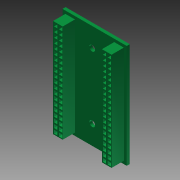
# Autodesk Inventor part: mbed breakout board
Saved by Autodesk Inventor 2012 (Build 160160000, 160)
## iProperties
Created: 2012-03-03
Part Number: mbed breakout board
Material: Default
Document SubType Name: Modeling
Designer: Lauszus
Density: 1 g/cm^3
Author: Lauszus
Autodesk Inventor part; units mm, degrees
ref_plane "YZ Plane" through (0, 0, 0) normal (1, 0, 0) x (0, 1, 0)
ref_plane "XZ Plane" through (0, 0, 0) normal (0, 1, 0) x (-1, 0, 0)
ref_plane "XY Plane" through (0, 0, 0) normal (0, 0, 1) x (1, 0, 0)
sketch "Sketch1" plane through (0, 0, 0) normal (0, 0, 1) x (1, 0, 0)
  line L0 (-20.4515, 31.3375) -> (12.9485, 31.3375)
  line L1 (12.9485, 31.3375) -> (12.9485, -22.6377)
  line L2 (12.9485, -22.6377) -> (-20.4515, -22.6377)
  line L3 (-20.4515, -22.6377) -> (-20.4515, 31.3375)
  line L4 (-18.9515, 29.8375) -> (-13.9515, 29.8375)
  line L5 (-13.9515, 29.8375) -> (-13.9515, -21.1377)
  line L6 (-13.9515, -21.1377) -> (-18.9515, -21.1377)
  line L7 (-18.9515, -21.1377) -> (-18.9515, 29.8375)
  line L8 (-18.4515, -20.6377) -> (-16.7515, -20.6377)
  line L9 (-16.7515, -20.6377) -> (-16.7515, -18.9377)
  line L10 (-16.7515, -18.9377) -> (-18.4515, -18.9377)
  line L11 (-18.4515, -18.9377) -> (-18.4515, -20.6377)
  line L12 (-15.9115, -20.6377) -> (-14.2115, -20.6377)
  line L13 (-14.2115, -20.6377) -> (-14.2115, -18.9377)
  line L14 (-14.2115, -18.9377) -> (-15.9115, -18.9377)
  line L15 (-15.9115, -18.9377) -> (-15.9115, -20.6377)
  line L16 (-18.4515, -18.0977) -> (-16.7515, -18.0977)
  line L17 (-16.7515, -18.0977) -> (-16.7515, -16.3977)
  line L18 (-16.7515, -16.3977) -> (-18.4515, -16.3977)
  line L19 (-18.4515, -16.3977) -> (-18.4515, -18.0977)
  line L20 (-15.9115, -18.0977) -> (-14.2115, -18.0977)
  line L21 (-14.2115, -18.0977) -> (-14.2115, -16.3977)
  line L22 (-14.2115, -16.3977) -> (-15.9115, -16.3977)
  line L23 (-15.9115, -16.3977) -> (-15.9115, -18.0977)
  line L24 (-18.4515, -15.5577) -> (-16.7515, -15.5577)
  line L25 (-16.7515, -15.5577) -> (-16.7515, -13.8577)
  line L26 (-16.7515, -13.8577) -> (-18.4515, -13.8577)
  line L27 (-18.4515, -13.8577) -> (-18.4515, -15.5577)
  line L28 (-15.9115, -15.5577) -> (-14.2115, -15.5577)
  line L29 (-14.2115, -15.5577) -> (-14.2115, -13.8577)
  line L30 (-14.2115, -13.8577) -> (-15.9115, -13.8577)
  line L31 (-15.9115, -13.8577) -> (-15.9115, -15.5577)
  line L32 (-14.2115, -11.3177) -> (-15.9115, -11.3177)
  line L33 (-14.2115, -13.0177) -> (-14.2115, -11.3177)
  line L34 (-15.9115, -11.3177) -> (-15.9115, -13.0177)
  line L35 (-15.9115, -13.0177) -> (-14.2115, -13.0177)
  line L36 (-18.4515, -13.0177) -> (-16.7515, -13.0177)
  line L37 (-16.7515, -13.0177) -> (-16.7515, -11.3177)
  line L38 (-16.7515, -11.3177) -> (-18.4515, -11.3177)
  line L39 (-18.4515, -11.3177) -> (-18.4515, -13.0177)
  line L40 (-18.4515, -10.4777) -> (-16.7515, -10.4777)
  line L41 (-16.7515, -10.4777) -> (-16.7515, -8.7777)
  line L42 (-16.7515, -8.7777) -> (-18.4515, -8.7777)
  line L43 (-18.4515, -8.7777) -> (-18.4515, -10.4777)
  line L44 (-15.9115, -10.4777) -> (-14.2115, -10.4777)
  line L45 (-14.2115, -10.4777) -> (-14.2115, -8.7777)
  line L46 (-14.2115, -8.7777) -> (-15.9115, -8.7777)
  line L47 (-15.9115, -8.7777) -> (-15.9115, -10.4777)
  line L48 (-14.2115, -6.2377) -> (-15.9115, -6.2377)
  line L49 (-14.2115, -7.9377) -> (-14.2115, -6.2377)
  line L50 (-15.9115, -6.2377) -> (-15.9115, -7.9377)
  line L51 (-15.9115, -7.9377) -> (-14.2115, -7.9377)
  line L52 (-18.4515, -7.9377) -> (-16.7515, -7.9377)
  line L53 (-16.7515, -7.9377) -> (-16.7515, -6.2377)
  line L54 (-16.7515, -6.2377) -> (-18.4515, -6.2377)
  line L55 (-18.4515, -6.2377) -> (-18.4515, -7.9377)
  line L56 (-18.4515, -5.3977) -> (-16.7515, -5.3977)
  line L57 (-16.7515, -5.3977) -> (-16.7515, -3.6977)
  line L58 (-16.7515, -3.6977) -> (-18.4515, -3.6977)
  line L59 (-18.4515, -3.6977) -> (-18.4515, -5.3977)
  line L60 (-15.9115, -5.3977) -> (-14.2115, -5.3977)
  line L61 (-14.2115, -5.3977) -> (-14.2115, -3.6977)
  line L62 (-14.2115, -3.6977) -> (-15.9115, -3.6977)
  line L63 (-15.9115, -3.6977) -> (-15.9115, -5.3977)
  line L64 (-14.2115, -1.1577) -> (-15.9115, -1.1577)
  line L65 (-14.2115, -2.8577) -> (-14.2115, -1.1577)
  line L66 (-15.9115, -1.1577) -> (-15.9115, -2.8577)
  line L67 (-15.9115, -2.8577) -> (-14.2115, -2.8577)
  line L68 (-18.4515, -2.8577) -> (-16.7515, -2.8577)
  line L69 (-16.7515, -2.8577) -> (-16.7515, -1.1577)
  line L70 (-16.7515, -1.1577) -> (-18.4515, -1.1577)
  line L71 (-18.4515, -1.1577) -> (-18.4515, -2.8577)
  line L72 (-18.4515, -0.3177) -> (-16.7515, -0.3177)
  line L73 (-16.7515, -0.3177) -> (-16.7515, 1.3823)
  line L74 (-16.7515, 1.3823) -> (-18.4515, 1.3823)
  line L75 (-18.4515, 1.3823) -> (-18.4515, -0.3177)
  line L76 (-15.9115, -0.3177) -> (-14.2115, -0.3177)
  line L77 (-14.2115, -0.3177) -> (-14.2115, 1.3823)
  line L78 (-14.2115, 1.3823) -> (-15.9115, 1.3823)
  line L79 (-15.9115, 1.3823) -> (-15.9115, -0.3177)
  line L80 (-14.2115, 3.9223) -> (-15.9115, 3.9223)
  line L81 (-14.2115, 2.2223) -> (-14.2115, 3.9223)
  line L82 (-15.9115, 3.9223) -> (-15.9115, 2.2223)
  line L83 (-15.9115, 2.2223) -> (-14.2115, 2.2223)
  line L84 (-18.4515, 2.2223) -> (-16.7515, 2.2223)
  line L85 (-16.7515, 2.2223) -> (-16.7515, 3.9223)
  line L86 (-16.7515, 3.9223) -> (-18.4515, 3.9223)
  line L87 (-18.4515, 3.9223) -> (-18.4515, 2.2223)
  line L88 (-18.4515, 4.7623) -> (-16.7515, 4.7623)
  line L89 (-16.7515, 4.7623) -> (-16.7515, 6.4623)
  line L90 (-16.7515, 6.4623) -> (-18.4515, 6.4623)
  line L91 (-18.4515, 6.4623) -> (-18.4515, 4.7623)
  line L92 (-15.9115, 4.7623) -> (-14.2115, 4.7623)
  line L93 (-14.2115, 4.7623) -> (-14.2115, 6.4623)
  line L94 (-14.2115, 6.4623) -> (-15.9115, 6.4623)
  line L95 (-15.9115, 6.4623) -> (-15.9115, 4.7623)
  line L96 (-14.2115, 9.0023) -> (-15.9115, 9.0023)
  line L97 (-14.2115, 7.3023) -> (-14.2115, 9.0023)
  line L98 (-15.9115, 9.0023) -> (-15.9115, 7.3023)
  line L99 (-15.9115, 7.3023) -> (-14.2115, 7.3023)
  line L100 (-18.4515, 7.3023) -> (-16.7515, 7.3023)
  line L101 (-16.7515, 7.3023) -> (-16.7515, 9.0023)
  line L102 (-16.7515, 9.0023) -> (-18.4515, 9.0023)
  line L103 (-18.4515, 9.0023) -> (-18.4515, 7.3023)
  line L104 (-18.4515, 9.8423) -> (-16.7515, 9.8423)
  line L105 (-16.7515, 9.8423) -> (-16.7515, 11.5423)
  line L106 (-16.7515, 11.5423) -> (-18.4515, 11.5423)
  line L107 (-18.4515, 11.5423) -> (-18.4515, 9.8423)
  line L108 (-15.9115, 9.8423) -> (-14.2115, 9.8423)
  line L109 (-14.2115, 9.8423) -> (-14.2115, 11.5423)
  line L110 (-14.2115, 11.5423) -> (-15.9115, 11.5423)
  line L111 (-15.9115, 11.5423) -> (-15.9115, 9.8423)
  line L112 (-14.2115, 14.0823) -> (-15.9115, 14.0823)
  line L113 (-14.2115, 12.3823) -> (-14.2115, 14.0823)
  line L114 (-15.9115, 14.0823) -> (-15.9115, 12.3823)
  line L115 (-15.9115, 12.3823) -> (-14.2115, 12.3823)
  line L116 (-18.4515, 12.3823) -> (-16.7515, 12.3823)
  line L117 (-16.7515, 12.3823) -> (-16.7515, 14.0823)
  line L118 (-16.7515, 14.0823) -> (-18.4515, 14.0823)
  line L119 (-18.4515, 14.0823) -> (-18.4515, 12.3823)
  line L120 (-18.4515, 14.9223) -> (-16.7515, 14.9223)
  line L121 (-16.7515, 14.9223) -> (-16.7515, 16.6223)
  line L122 (-16.7515, 16.6223) -> (-18.4515, 16.6223)
  line L123 (-18.4515, 16.6223) -> (-18.4515, 14.9223)
  line L124 (-15.9115, 14.9223) -> (-14.2115, 14.9223)
  line L125 (-14.2115, 14.9223) -> (-14.2115, 16.6223)
  line L126 (-14.2115, 16.6223) -> (-15.9115, 16.6223)
  line L127 (-15.9115, 16.6223) -> (-15.9115, 14.9223)
  line L128 (-14.2115, 19.1623) -> (-15.9115, 19.1623)
  line L129 (-14.2115, 17.4623) -> (-14.2115, 19.1623)
  line L130 (-15.9115, 19.1623) -> (-15.9115, 17.4623)
  line L131 (-15.9115, 17.4623) -> (-14.2115, 17.4623)
  line L132 (-18.4515, 17.4623) -> (-16.7515, 17.4623)
  line L133 (-16.7515, 17.4623) -> (-16.7515, 19.1623)
  line L134 (-16.7515, 19.1623) -> (-18.4515, 19.1623)
  line L135 (-18.4515, 19.1623) -> (-18.4515, 17.4623)
  line L136 (-18.4515, 20.0023) -> (-16.7515, 20.0023)
  line L137 (-16.7515, 20.0023) -> (-16.7515, 21.7023)
  line L138 (-16.7515, 21.7023) -> (-18.4515, 21.7023)
  line L139 (-18.4515, 21.7023) -> (-18.4515, 20.0023)
  line L140 (-15.9115, 20.0023) -> (-14.2115, 20.0023)
  line L141 (-14.2115, 20.0023) -> (-14.2115, 21.7023)
  line L142 (-14.2115, 21.7023) -> (-15.9115, 21.7023)
  line L143 (-15.9115, 21.7023) -> (-15.9115, 20.0023)
  line L144 (-14.2115, 24.2423) -> (-15.9115, 24.2423)
  line L145 (-14.2115, 22.5423) -> (-14.2115, 24.2423)
  line L146 (-15.9115, 24.2423) -> (-15.9115, 22.5423)
  line L147 (-15.9115, 22.5423) -> (-14.2115, 22.5423)
  line L148 (-18.4515, 22.5423) -> (-16.7515, 22.5423)
  line L149 (-16.7515, 22.5423) -> (-16.7515, 24.2423)
  line L150 (-16.7515, 24.2423) -> (-18.4515, 24.2423)
  line L151 (-18.4515, 24.2423) -> (-18.4515, 22.5423)
  line L152 (-18.4515, 25.0823) -> (-16.7515, 25.0823)
  line L153 (-16.7515, 25.0823) -> (-16.7515, 26.7823)
  line L154 (-16.7515, 26.7823) -> (-18.4515, 26.7823)
  line L155 (-18.4515, 26.7823) -> (-18.4515, 25.0823)
  line L156 (-15.9115, 25.0823) -> (-14.2115, 25.0823)
  line L157 (-14.2115, 25.0823) -> (-14.2115, 26.7823)
  line L158 (-14.2115, 26.7823) -> (-15.9115, 26.7823)
  line L159 (-15.9115, 26.7823) -> (-15.9115, 25.0823)
  line L160 (-14.2115, 29.3223) -> (-15.9115, 29.3223)
  line L161 (-14.2115, 27.6223) -> (-14.2115, 29.3223)
  line L162 (-15.9115, 29.3223) -> (-15.9115, 27.6223)
  line L163 (-15.9115, 27.6223) -> (-14.2115, 27.6223)
  line L164 (-18.4515, 27.6223) -> (-16.7515, 27.6223)
  line L165 (-16.7515, 27.6223) -> (-16.7515, 29.3223)
  line L166 (-16.7515, 29.3223) -> (-18.4515, 29.3223)
  line L167 (-18.4515, 29.3223) -> (-18.4515, 27.6223)
  line L168 (6.4485, 29.8375) -> (11.4485, 29.8375)
  line L169 (11.4485, 29.8375) -> (11.4485, -21.1377)
  line L170 (11.4485, -21.1377) -> (6.4485, -21.1377)
  line L171 (6.4485, -21.1377) -> (6.4485, 29.8375)
  line L172 (6.9485, -20.6377) -> (8.6485, -20.6377)
  line L173 (8.6485, -20.6377) -> (8.6485, -18.9377)
  line L174 (8.6485, -18.9377) -> (6.9485, -18.9377)
  line L175 (6.9485, -18.9377) -> (6.9485, -20.6377)
  line L176 (9.4885, -20.6377) -> (11.1885, -20.6377)
  line L177 (11.1885, -20.6377) -> (11.1885, -18.9377)
  line L178 (11.1885, -18.9377) -> (9.4885, -18.9377)
  line L179 (9.4885, -18.9377) -> (9.4885, -20.6377)
  line L180 (11.1885, -16.3977) -> (9.4885, -16.3977)
  line L181 (11.1885, -18.0977) -> (11.1885, -16.3977)
  line L182 (9.4885, -16.3977) -> (9.4885, -18.0977)
  line L183 (9.4885, -18.0977) -> (11.1885, -18.0977)
  line L184 (6.9485, -18.0977) -> (8.6485, -18.0977)
  line L185 (8.6485, -18.0977) -> (8.6485, -16.3977)
  line L186 (8.6485, -16.3977) -> (6.9485, -16.3977)
  line L187 (6.9485, -16.3977) -> (6.9485, -18.0977)
  line L188 (6.9485, -15.5577) -> (8.6485, -15.5577)
  line L189 (6.9485, -13.8577) -> (6.9485, -15.5577)
  line L190 (8.6485, -13.8577) -> (6.9485, -13.8577)
  line L191 (8.6485, -15.5577) -> (8.6485, -13.8577)
  line L192 (6.9485, -13.0177) -> (8.6485, -13.0177)
  line L193 (6.9485, -11.3177) -> (6.9485, -13.0177)
  line L194 (8.6485, -11.3177) -> (6.9485, -11.3177)
  line L195 (8.6485, -13.0177) -> (8.6485, -11.3177)
  line L196 (11.1885, -11.3177) -> (9.4885, -11.3177)
  line L197 (9.4885, -11.3177) -> (9.4885, -13.0177)
  line L198 (11.1885, -13.0177) -> (11.1885, -11.3177)
  line L199 (9.4885, -13.0177) -> (11.1885, -13.0177)
  line L200 (11.1885, -13.8577) -> (9.4885, -13.8577)
  line L201 (9.4885, -13.8577) -> (9.4885, -15.5577)
  line L202 (9.4885, -15.5577) -> (11.1885, -15.5577)
  line L203 (11.1885, -15.5577) -> (11.1885, -13.8577)
  line L204 (6.9485, -10.4777) -> (8.6485, -10.4777)
  line L205 (6.9485, -8.7777) -> (6.9485, -10.4777)
  line L206 (8.6485, -8.7777) -> (6.9485, -8.7777)
  line L207 (8.6485, -10.4777) -> (8.6485, -8.7777)
  line L208 (6.9485, -7.9377) -> (8.6485, -7.9377)
  line L209 (6.9485, -6.2377) -> (6.9485, -7.9377)
  line L210 (8.6485, -6.2377) -> (6.9485, -6.2377)
  line L211 (8.6485, -7.9377) -> (8.6485, -6.2377)
  line L212 (11.1885, -6.2377) -> (9.4885, -6.2377)
  line L213 (9.4885, -6.2377) -> (9.4885, -7.9377)
  line L214 (11.1885, -7.9377) -> (11.1885, -6.2377)
  line L215 (9.4885, -7.9377) -> (11.1885, -7.9377)
  line L216 (11.1885, -8.7777) -> (9.4885, -8.7777)
  line L217 (9.4885, -8.7777) -> (9.4885, -10.4777)
  line L218 (9.4885, -10.4777) -> (11.1885, -10.4777)
  line L219 (11.1885, -10.4777) -> (11.1885, -8.7777)
  line L220 (6.9485, -5.3977) -> (8.6485, -5.3977)
  line L221 (6.9485, -3.6977) -> (6.9485, -5.3977)
  line L222 (8.6485, -3.6977) -> (6.9485, -3.6977)
  line L223 (8.6485, -5.3977) -> (8.6485, -3.6977)
  line L224 (6.9485, -2.8577) -> (8.6485, -2.8577)
  line L225 (6.9485, -1.1577) -> (6.9485, -2.8577)
  line L226 (8.6485, -1.1577) -> (6.9485, -1.1577)
  line L227 (8.6485, -2.8577) -> (8.6485, -1.1577)
  line L228 (11.1885, -1.1577) -> (9.4885, -1.1577)
  line L229 (9.4885, -1.1577) -> (9.4885, -2.8577)
  line L230 (11.1885, -2.8577) -> (11.1885, -1.1577)
  line L231 (9.4885, -2.8577) -> (11.1885, -2.8577)
  line L232 (11.1885, -3.6977) -> (9.4885, -3.6977)
  line L233 (9.4885, -3.6977) -> (9.4885, -5.3977)
  line L234 (9.4885, -5.3977) -> (11.1885, -5.3977)
  line L235 (11.1885, -5.3977) -> (11.1885, -3.6977)
  line L236 (6.9485, -0.3177) -> (8.6485, -0.3177)
  line L237 (6.9485, 1.3823) -> (6.9485, -0.3177)
  line L238 (8.6485, 1.3823) -> (6.9485, 1.3823)
  line L239 (8.6485, -0.3177) -> (8.6485, 1.3823)
  line L240 (6.9485, 2.2223) -> (8.6485, 2.2223)
  line L241 (6.9485, 3.9223) -> (6.9485, 2.2223)
  line L242 (8.6485, 3.9223) -> (6.9485, 3.9223)
  line L243 (8.6485, 2.2223) -> (8.6485, 3.9223)
  line L244 (11.1885, 3.9223) -> (9.4885, 3.9223)
  line L245 (9.4885, 3.9223) -> (9.4885, 2.2223)
  line L246 (11.1885, 2.2223) -> (11.1885, 3.9223)
  line L247 (9.4885, 2.2223) -> (11.1885, 2.2223)
  line L248 (11.1885, 1.3823) -> (9.4885, 1.3823)
  line L249 (9.4885, 1.3823) -> (9.4885, -0.3177)
  line L250 (9.4885, -0.3177) -> (11.1885, -0.3177)
  line L251 (11.1885, -0.3177) -> (11.1885, 1.3823)
  line L252 (6.9485, 4.7623) -> (8.6485, 4.7623)
  line L253 (6.9485, 6.4623) -> (6.9485, 4.7623)
  line L254 (8.6485, 6.4623) -> (6.9485, 6.4623)
  line L255 (8.6485, 4.7623) -> (8.6485, 6.4623)
  line L256 (6.9485, 7.3023) -> (8.6485, 7.3023)
  line L257 (6.9485, 9.0023) -> (6.9485, 7.3023)
  line L258 (8.6485, 9.0023) -> (6.9485, 9.0023)
  line L259 (8.6485, 7.3023) -> (8.6485, 9.0023)
  line L260 (11.1885, 9.0023) -> (9.4885, 9.0023)
  line L261 (9.4885, 9.0023) -> (9.4885, 7.3023)
  line L262 (11.1885, 7.3023) -> (11.1885, 9.0023)
  line L263 (9.4885, 7.3023) -> (11.1885, 7.3023)
  line L264 (11.1885, 6.4623) -> (9.4885, 6.4623)
  line L265 (9.4885, 6.4623) -> (9.4885, 4.7623)
  line L266 (9.4885, 4.7623) -> (11.1885, 4.7623)
  line L267 (11.1885, 4.7623) -> (11.1885, 6.4623)
  line L268 (6.9485, 9.8423) -> (8.6485, 9.8423)
  line L269 (6.9485, 11.5423) -> (6.9485, 9.8423)
  line L270 (8.6485, 11.5423) -> (6.9485, 11.5423)
  line L271 (8.6485, 9.8423) -> (8.6485, 11.5423)
  line L272 (6.9485, 12.3823) -> (8.6485, 12.3823)
  line L273 (6.9485, 14.0823) -> (6.9485, 12.3823)
  line L274 (8.6485, 14.0823) -> (6.9485, 14.0823)
  line L275 (8.6485, 12.3823) -> (8.6485, 14.0823)
  line L276 (11.1885, 14.0823) -> (9.4885, 14.0823)
  line L277 (9.4885, 14.0823) -> (9.4885, 12.3823)
  line L278 (11.1885, 12.3823) -> (11.1885, 14.0823)
  line L279 (9.4885, 12.3823) -> (11.1885, 12.3823)
  line L280 (11.1885, 11.5423) -> (9.4885, 11.5423)
  line L281 (9.4885, 11.5423) -> (9.4885, 9.8423)
  line L282 (9.4885, 9.8423) -> (11.1885, 9.8423)
  line L283 (11.1885, 9.8423) -> (11.1885, 11.5423)
  line L284 (6.9485, 14.9223) -> (8.6485, 14.9223)
  line L285 (6.9485, 16.6223) -> (6.9485, 14.9223)
  line L286 (8.6485, 16.6223) -> (6.9485, 16.6223)
  line L287 (8.6485, 14.9223) -> (8.6485, 16.6223)
  line L288 (6.9485, 17.4623) -> (8.6485, 17.4623)
  line L289 (6.9485, 19.1623) -> (6.9485, 17.4623)
  line L290 (8.6485, 19.1623) -> (6.9485, 19.1623)
  line L291 (8.6485, 17.4623) -> (8.6485, 19.1623)
  line L292 (11.1885, 19.1623) -> (9.4885, 19.1623)
  line L293 (9.4885, 19.1623) -> (9.4885, 17.4623)
  line L294 (11.1885, 17.4623) -> (11.1885, 19.1623)
  line L295 (9.4885, 17.4623) -> (11.1885, 17.4623)
  line L296 (11.1885, 16.6223) -> (9.4885, 16.6223)
  line L297 (9.4885, 16.6223) -> (9.4885, 14.9223)
  line L298 (9.4885, 14.9223) -> (11.1885, 14.9223)
  line L299 (11.1885, 14.9223) -> (11.1885, 16.6223)
  line L300 (6.9485, 20.0023) -> (8.6485, 20.0023)
  line L301 (6.9485, 21.7023) -> (6.9485, 20.0023)
  line L302 (8.6485, 21.7023) -> (6.9485, 21.7023)
  line L303 (8.6485, 20.0023) -> (8.6485, 21.7023)
  line L304 (6.9485, 22.5423) -> (8.6485, 22.5423)
  line L305 (6.9485, 24.2423) -> (6.9485, 22.5423)
  line L306 (8.6485, 24.2423) -> (6.9485, 24.2423)
  line L307 (8.6485, 22.5423) -> (8.6485, 24.2423)
  line L308 (11.1885, 24.2423) -> (9.4885, 24.2423)
  line L309 (9.4885, 24.2423) -> (9.4885, 22.5423)
  line L310 (11.1885, 22.5423) -> (11.1885, 24.2423)
  line L311 (9.4885, 22.5423) -> (11.1885, 22.5423)
  line L312 (11.1885, 21.7023) -> (9.4885, 21.7023)
  line L313 (9.4885, 21.7023) -> (9.4885, 20.0023)
  line L314 (9.4885, 20.0023) -> (11.1885, 20.0023)
  line L315 (11.1885, 20.0023) -> (11.1885, 21.7023)
  line L316 (6.9485, 25.0823) -> (8.6485, 25.0823)
  line L317 (6.9485, 26.7823) -> (6.9485, 25.0823)
  line L318 (8.6485, 26.7823) -> (6.9485, 26.7823)
  line L319 (8.6485, 25.0823) -> (8.6485, 26.7823)
  line L320 (6.9485, 27.6223) -> (8.6485, 27.6223)
  line L321 (6.9485, 29.3223) -> (6.9485, 27.6223)
  line L322 (8.6485, 29.3223) -> (6.9485, 29.3223)
  line L323 (8.6485, 27.6223) -> (8.6485, 29.3223)
  line L324 (11.1885, 29.3223) -> (9.4885, 29.3223)
  line L325 (9.4885, 29.3223) -> (9.4885, 27.6223)
  line L326 (11.1885, 27.6223) -> (11.1885, 29.3223)
  line L327 (9.4885, 27.6223) -> (11.1885, 27.6223)
  line L328 (11.1885, 26.7823) -> (9.4885, 26.7823)
  line L329 (9.4885, 26.7823) -> (9.4885, 25.0823)
  line L330 (9.4885, 25.0823) -> (11.1885, 25.0823)
  line L331 (11.1885, 25.0823) -> (11.1885, 26.7823)
  circle A0 centre (-5.0215, 21.3375) radius 1.5
  circle A1 centre (-5.0215, -12.6377) radius 1.5
  point P0 (0, 0)
  dimension "d3" = 50.9753
  dimension "d4" = 5
  dimension "d5" = 1.5
  dimension "d6" = 1.5
  dimension "d7" = 1.7
  dimension "d8" = 1.7
  dimension "d9" = 2.54
  dimension "d10" = 1.7
  dimension "d11" = 1.7
  dimension "d12" = 0.5
  dimension "d13" = 0.5
  dimension "d14" = 0.5
  dimension "d15" = 1.7
  dimension "d16" = 1.7
  dimension "d17" = 2.54
  dimension "d18" = 1.7
  dimension "d19" = 1.7
  dimension "d21" = 2.54
  dimension "d22" = 2.54
  dimension "d23" = 0.5
  dimension "d26" = 5.08
  dimension "d33" = 25.4
  dimension "d38" = 1.5
  dimension "d39" = 1.5
  dimension "d40" = 15.43
  dimension "d41" = 15.43
  dimension "d42" = 10
  dimension "d43" = 10
  dimension "d44" = 3
  dimension "d45" = 3
  constraints: 664 end point, 12 parallel, 7 horizontal, 6 perpendicular, 2 centre point, 1 vertical, 616 other
  measures "d3" distance of L4.end L5.end
  measures "d4" distance of L4.start L4.end
  measures "d5" distance between parallel lines of L2 L6
  measures "d6" distance between parallel lines of L3 L7
  measures "d7" distance of L10.end L8.start
  measures "d8" distance of L9.end L10.end
  measures "d9" distance between parallel lines of L11 L15
  measures "d10" distance of L14.end L12.start
  measures "d11" distance of L13.end L14.end
  measures "d12" distance between parallel lines of L7 L11
  measures "d13" distance between parallel lines of L6 L8
  measures "d14" distance between parallel lines of L6 L12
  measures "d15" distance of L18.end L16.start
  measures "d16" distance of L17.end L18.end
  measures "d17" distance between parallel lines of L19 L23
  measures "d18" distance of L22.end L23.end
  measures "d19" distance of L22.start L22.end
  measures "d21" distance between parallel lines of L8 L16
  measures "d22" distance between parallel lines of L12 L20
  measures "d23" distance between parallel lines of L7 L19
  measures "d26" distance of L8.start L24.start
  measures "d33" distance of L27.start L189.start
  measures "d38" distance between parallel lines of L1 L169
  measures "d39" distance between parallel lines of L4 L0
  measures "d40" distance from line of L3 A0.centre
  measures "d41" distance from line of L3 A1.centre
  measures "d42" distance from line of L0 A0.centre
  measures "d43" distance from line of A1.centre L2
  measures "d44" diameter of A0
  measures "d45" diameter of A1
extrude "Extrusion1" add sketch "Sketch1" along normal blind 1.6 contours L0 L1 L2 L3 | L4 L5 L6 L7 | L11 L10 L9 L8 | L15 L14 L13 L12 | L19 L18 L17 L16 | L23 L22 L21 L20 | L27 L26 L25 L24 | L31 L30 L29 L28 | L33 L35 L34 L32 | L39 L38 L37 L36 | L43 L42 L41 L40 | L47 L46 L45 L44 | L49 L51 L50 L48 | L55 L54 L53 L52 | L59 L58 L57 L56 | L63 L62 L61 L60 | L65 L67 L66 L64 | L71 L70 L69 L68 | L75 L74 L73 L72 | L79 L78 L77 L76 | L81 L83 L82 L80 | L87 L86 L85 L84 | L91 L90 L89 L88 | L95 L94 L93 L92 | L97 L99 L98 L96 | L103 L102 L101 L100 | L107 L106 L105 L104 | L111 L110 L109 L108 | L113 L115 L114 L112 | L119 L118 L117 L116 | L123 L122 L121 L120 | L127 L126 L125 L124 | L129 L131 L130 L128 | L135 L134 L133 L132 | L139 L138 L137 L136 | L143 L142 L141 L140 | L145 L147 L146 L144 | L151 L150 L149 L148 | L155 L154 L153 L152 | L159 L158 L157 L156 | L161 L163 L162 L160 | L167 L166 L165 L164 | L168 L169 L170 L171 | L175 L174 L173 L172 | L179 L178 L177 L176 | L181 L183 L182 L180 | L187 L186 L185 L184 | L189 L190 L191 L188 | L193 L194 L195 L192 | L198 L199 L197 L196 | L203 L202 L201 L200 | L205 L206 L207 L204 | L209 L210 L211 L208 | L214 L215 L213 L212 | L219 L218 L217 L216 | L221 L222 L223 L220 | L225 L226 L227 L224 | L230 L231 L229 L228 | L235 L234 L233 L232 | L237 L238 L239 L236 | L241 L242 L243 L240 | L246 L247 L245 L244 | L251 L250 L249 L248 | L253 L254 L255 L252 | L257 L258 L259 L256 | L262 L263 L261 L260 | L267 L266 L265 L264 | L269 L270 L271 L268 | L273 L274 L275 L272 | L278 L279 L277 L276 | L283 L282 L281 L280 | L285 L286 L287 L284 | L289 L290 L291 L288 | L294 L295 L293 L292 | L299 L298 L297 L296 | L301 L302 L303 L300 | L305 L306 L307 L304 | L310 L311 L309 L308 | L315 L314 L313 L312 | L317 L318 L319 L316 | L321 L322 L323 L320 | L326 L327 L325 L324 | L331 L330 L329 L328
extrude "Extrusion2" add sketch "Sketch1" along normal blind 8 contours L4 L5 L6 L7 | L168 L169 L170 L171
body "Solid1"
